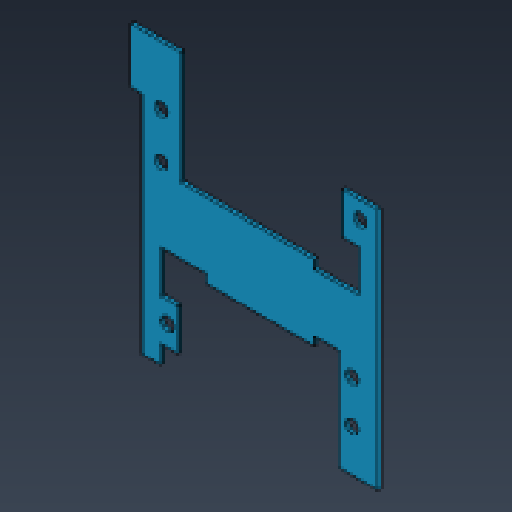
# Autodesk Inventor part: PCB_interface
Saved by Autodesk Inventor 2026.2 (Build 302298010, 298A)
## iProperties
Created: 2026-04-04
Part Number: PCB_interface
Material: Generic
Document SubType Name: Modeling
Designer: szymo
Density: 1 g/cm^3
Appearance: Default(1)
Author: szymo
Autodesk Inventor part; units mm, degrees
ref_plane "YZ Plane" through (0, 0, 0) normal (1, 0, 0) x (0, 1, 0)
ref_plane "XZ Plane" through (0, 0, 0) normal (0, 1, 0) x (-1, 0, 0)
ref_plane "XY Plane" through (0, 0, 0) normal (0, 0, 1) x (1, 0, 0)
sketch "Sketch1" plane through (0, 0, 0) normal (0, 0, 1) x (1, 0, 0)
  line L0 (0, 0) -> (0, 9.8085) projected
  line L1 (0, 9.8085) -> (-4, 9.8085) projected
  line L2 (-4, 9.8085) -> (-4, 14.7474) projected
  line L3 (0, 14.7474) -> (-4, 14.7474) projected
  line L4 (0, 14.7474) -> (0, 16.5483) projected
  line L5 (0, 16.5483) -> (0.6, 16.5483) projected
  line L6 (0.6, 61.0677) -> (0.6, 16.5483) projected
  line L7 (0.6, 61.0677) -> (-8.5, 61.0677) projected
  line L8 (-8.5, -4.2282) -> (-8.5, 61.0677) projected
  line L9 (0, -4.2282) -> (-8.5, -4.2282) projected
  line L10 (0, -4.2282) -> (0, -4.0158) projected
  line L11 (0, -4.0158) -> (-4, -4.0158) projected
  line L12 (-4, -4.0158) -> (-4, 0) projected
  line L13 (0, 0) -> (-4, 0) projected
  line L14 (38, 42.531) -> (38, 52.3395) projected
  line L15 (38, 42.531) -> (42, 42.531) projected
  line L16 (42, 37.5922) -> (42, 42.531) projected
  line L17 (38, 37.5922) -> (42, 37.5922) projected
  line L18 (38, 35.7912) -> (38, 37.5922) projected
  line L19 (38, 35.7912) -> (37.4, 35.7912) projected
  line L20 (37.4, -4.2282) -> (37.4, 35.7912) projected
  line L21 (46.5, -4.2282) -> (37.4, -4.2282) projected
  line L22 (46.5, 61.0677) -> (46.5, -4.2282) projected
  line L23 (46.5, 61.0677) -> (37.4, 61.0677) projected
  line L24 (37.4, 57.3442) -> (37.4, 61.0677) projected
  line L25 (38, 57.3442) -> (37.4, 57.3442) projected
  line L26 (38, 56.3553) -> (38, 57.3442) projected
  line L27 (38, 56.3553) -> (42, 56.3553) projected
  line L28 (42, 52.3395) -> (42, 56.3553) projected
  line L29 (38, 52.3395) -> (42, 52.3395) projected
  line L30 (0, 16.5483) -> (37.4, 16.5483)
  line L31 (37.4, 16.5483) -> (37.4, -5.0046)
  line L32 (37.4, -5.0046) -> (0, -5.0046)
  line L33 (0, -5.0046) -> (0, 11.1139)
  line L34 (0, 11.1139) -> (-3, 11.1139)
  line L35 (-3, 11.1139) -> (-3, 13.2925)
  line L36 (-3, 13.2925) -> (0, 13.2925)
  line L37 (0, 13.2925) -> (0, 16.5483)
  line L38 (5.5, 17.3718) -> (33.4, 17.3718)
  line L39 (33.4, 17.3718) -> (33.4, 16.5483)
  line L40 (33.4, 16.5483) -> (5.5, 16.5483)
  line L41 (5.5, 16.5483) -> (5.5, 17.3718)
  line L42 (33.4, -5.8282) -> (5.5, -5.8282)
  line L43 (5.5, -5.8282) -> (5.5, -5.0046)
  line L44 (5.5, -5.0046) -> (33.4, -5.0046)
  line L45 (33.4, -5.0046) -> (33.4, -5.8282)
  line L46 (32.5, 34.9677) -> (4.6, 34.9677)
  line L47 (4.6, 34.9677) -> (4.6, 35.7912)
  line L48 (4.6, 35.7912) -> (32.5, 35.7912)
  line L49 (32.5, 35.7912) -> (32.5, 34.9677)
  line L50 (4.6, 58.1677) -> (32.5, 58.1677)
  line L51 (32.5, 58.1677) -> (32.5, 57.3442)
  line L52 (32.5, 57.3442) -> (4.6, 57.3442)
  line L53 (4.6, 57.3442) -> (4.6, 58.1677)
  line L54 (38, 35.7912) -> (0.6, 35.7912)
  line L55 (0.6, 35.7912) -> (0.6, 57.3442)
  line L56 (0.6, 57.3442) -> (38, 57.3442)
  line L57 (38, 57.3442) -> (38, 41.2256)
  line L58 (38, 41.2256) -> (41, 41.2256)
  line L59 (41, 41.2256) -> (41, 39.047)
  line L60 (41, 39.047) -> (38, 39.047)
  line L61 (38, 39.047) -> (38, 35.7912)
  line L62 (0.6, 61.0677) -> (0.6, 33.5519)
  line L63 (0.5, 60.9677) -> (0.5, 34.8677)
  line L64 (0.5, 34.8677) -> (31.5, 34.8677)
  line L65 (0.5, 60.9677) -> (-8.4, 60.9677)
  line L66 (31.5, 34.8677) -> (31.5, 32.8677)
  line L67 (46.4, 32.8669) -> (46.4, -4.1282)
  line L68 (46.4, -4.1282) -> (37.5, -4.1282)
  line L69 (37.5, -4.1282) -> (37.5, 19.4718)
  line L70 (37.5, 19.4718) -> (31.5, 19.4718)
  line L71 (31.5, 19.4718) -> (31.5, 17.4718)
  line L72 (31.5, 17.4718) -> (27.7928, 17.4718)
  line L73 (27.7928, 17.4718) -> (6.5, 17.4718)
  line L74 (6.5, 17.4718) -> (6.5, 19.4718)
  line L75 (6.5, 19.4718) -> (-4.1, 19.4718)
  line L76 (-4.1, -4.1282) -> (-8.4, -4.1282)
  line L77 (-8.4, -4.1282) -> (-8.4, 60.9677)
  line L78 (31.5, 32.8677) -> (42.1, 32.8677)
  line L79 (42.1013, 60.9677) -> (46.4, 60.9677)
  line L80 (46.4, 60.9677) -> (46.4, 32.8669)
  line L81 (42.1, 32.8677) -> (42.1, 42.631)
  line L82 (42.1, 42.631) -> (38.1, 42.631)
  line L83 (38.1, 42.631) -> (38.1, 52.2395)
  line L84 (38.1, 52.2395) -> (42.1, 52.2395)
  line L85 (42.1, 52.2395) -> (42.1, 57.4442)
  line L86 (42.1, 57.4442) -> (37.5, 57.4442)
  line L87 (37.5, 57.4442) -> (37.5, 60.9677)
  line L88 (37.5, 60.9677) -> (42.1013, 60.9677)
  line L89 (-4.1, 19.4718) -> (-4.1, 9.7085)
  line L90 (-4.1, 9.7085) -> (-0.1, 9.7085)
  line L91 (-0.1, 9.7085) -> (-0.1, 0.1)
  line L92 (-0.1, 0.1) -> (-4.1, 0.1)
  line L93 (-4.1, 0.1) -> (-4.1, -4.1282)
  circle A0 centre (-2.5, 4.9042) radius 2.25 projected
  circle A1 centre (-3.95, 36.6898) radius 2.25 projected
  circle A2 centre (-3.95, 47.2465) radius 2.25 projected
  circle A3 centre (43.8, 58.3677) radius 2.25 projected
  circle A4 centre (40.4, 5.6641) radius 2.25 projected
  circle A5 centre (40.4, 15.5803) radius 2.25 projected
  circle A6 centre (42.25, 48.1395) radius 2.25 projected
  line L94 (42.1, 52.2395) -> (46.4, 52.2395)
  line L95 (-8.5, 61.0677) -> (-8.5, 48.0677) projected
  line L96 (-8.5, 61.0677) -> (-17, 61.0677) projected
  line L97 (-17, 56.3177) -> (-17, 61.0677) projected
  line L98 (-11.2, 56.3177) -> (-17, 56.3177) projected
  line L99 (-11.2, 56.3177) -> (-11.2, 48.0677) projected
  line L100 (-8.5, 48.0677) -> (-11.2, 48.0677) projected
  line L101 (-8.4, 60.9677) -> (-11.1, 60.9677)
  line L102 (-11.1, 60.9677) -> (-11.1, 48.1677)
  line L103 (-11.1, 48.1677) -> (-8.4, 48.1677)
  dimension "d0" = 0.1
  dimension "d1" = 0.1
  dimension "d2" = 0.1
  dimension "d5" = 0.1
  dimension "d6" = 0.1
  dimension "d7" = 0.1
  dimension "d8" = 6
  dimension "d9" = 2
  dimension "d10" = 6
  dimension "d12" = 0.1
  dimension "d13" = 2
  dimension "d14" = 6
  dimension "d15" = 0.1
  dimension "d17" = 0.1
  dimension "d18" = 2
  dimension "d20" = 0.1
  dimension "d21" = 0.1
  dimension "d22" = 0.1
  dimension "d23" = 0.1
  dimension "d24" = 0.1
  dimension "d25" = 0.1
  dimension "d26" = 0.1
  dimension "d27" = 0.1
  dimension "d28" = 0.1
  dimension "d29" = 0.1
  dimension "d30" = 0.1
  dimension "d41" = 11.6
  dimension "d42" = 0.1
  dimension "d45" = 0.1
  dimension "d46" = 0
  constraints: 136 end point, 27 vertical, 22 horizontal, 14 perpendicular, 7 point on line, 2 parallel, 29 other
  measures "d0" distance between parallel lines of L64 L46
  measures "d1" distance between parallel lines of L6 L63
  measures "d2" distance between parallel lines of L7 L65
  measures "d5" distance between parallel lines of L22 L67
  measures "d6" distance between parallel lines of L21 L68
  measures "d7" distance between parallel lines of L20 L69
  measures "d8" distance between parallel lines of L69 L71
  measures "d9" distance between parallel lines of L72 L70
  measures "d10" distance between parallel lines of L69 L66
  measures "d12" distance between parallel lines of L38 L72
  measures "d13" distance between parallel lines of L75 L73
  measures "d14" distance between parallel lines of L63 L74
  measures "d15" distance between parallel lines of L77 L8
  measures "d17" distance between parallel lines of L9 L76
  measures "d18" distance between parallel lines of L64 L78
  measures "d20" distance between parallel lines of L23 L88
  measures "d21" distance between parallel lines of L24 L87
  measures "d22" distance between parallel lines of L25 L86
  measures "d23" distance between parallel lines of L28 L85
  measures "d24" distance between parallel lines of L29 L84
  measures "d25" distance between parallel lines of L14 L83
  measures "d26" distance between parallel lines of L82 L15
  measures "d27" distance between parallel lines of L93 L12
  measures "d28" distance between parallel lines of L92 L13
  measures "d29" distance between parallel lines of L0 L91
  measures "d30" distance between parallel lines of L1 L90
  measures "d41" distance between parallel lines of L63 L102
  measures "d42" distance between parallel lines of L102 L99
  measures "d45" distance between parallel lines of L103 L100
  measures "d46" distance between parallel lines of L84 L94
extrude "Extrusion1" add sketch "Sketch1" along normal blind 0.8 contours L103 L102 L101 L8 | L8 L101 L77 L103 | L77 L65 L63 L64 L6 L75 L89 L90 L91 L92 L93 L76 | L6 L64 L66 L78 L20 L70 L71 L72 L73 L74 L75 | L20 L78 L81 L82 L83 L84 L94 L80 L67 L68 L69 L70 | A0 | A1 | A2 | A4 | A5 | A6
hole "Hole1" at (-3.95, 47.2465, 0) at (-3.95, 36.6898, 0) at (-2.5, 4.9042, 0) at (40.4, 5.6641, 0) at (40.4, 15.5803, 0) at (42.25, 48.1395, 0) direction (0, 0, 1) diameter 3 end through all
body "Solid1"
